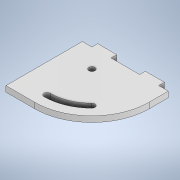
# Autodesk Inventor part: camMount
Saved by Autodesk Inventor 2020 (Build 240168000, 168)
## iProperties
Created: 2019-08-06
Part Number: camMount
Material: Generic
Document SubType Name: Modeling
Designer: n10208577
Density: 1 g/cm^3
Appearance: Default
Author: n10208577
Autodesk Inventor part; units mm, degrees
ref_plane "YZ Plane" through (0, 0, 0) normal (1, 0, 0) x (0, 1, 0)
ref_plane "XZ Plane" through (0, 0, 0) normal (0, 1, 0) x (-1, 0, 0)
ref_plane "XY Plane" through (0, 0, 0) normal (0, 0, 1) x (1, 0, 0)
sketch "Sketch1" plane through (0, 0, 0) normal (0, 1, 0) x (-1, 0, 0)
  arc A0 (9.7034, 16.3774) -> (9.7034, 19.5774) centre (9.7034, 17.9774) ccw
  circle A1 centre (9.7034, -5.5226) radius 1.6
  line L0 (9.7034, -15.5226) -> (-5.2966, -15.5226)
  line L1 (-15.2966, -15.5226) -> (-20.2966, -15.5226)
  line L2 (19.7034, -15.5226) -> (24.7034, -15.5226)
  line L3 (24.7034, -15.5226) -> (24.7034, 24.4774)
  line L4 (24.7034, 24.4774) -> (9.7034, 24.4774)
  arc A2 (-8.0449, 12.2258) -> (-5.7822, 9.963) centre (-6.9136, 11.0944) ccw
  arc A3 (9.7034, 16.3774) -> (-5.7822, 9.963) centre (9.7034, -5.5226) ccw
  arc A4 (9.7034, 19.5774) -> (-8.0449, 12.2258) centre (9.7034, -5.5226) ccw
  arc A5 (9.7034, 24.4774) -> (-20.2966, -5.5226) centre (9.7034, -5.5226) ccw
  line L5 (-20.2966, -15.5226) -> (-20.2966, -5.5226)
  line L6 (-15.2966, -15.5226) -> (-15.2966, -18.5226)
  line L7 (-15.2966, -18.5226) -> (-5.2966, -18.5226)
  line L8 (-5.2966, -18.5226) -> (-5.2966, -15.5226)
  line L9 (24.7034, -15.5226) -> (19.7034, -15.5226)
  line L10 (19.7034, -15.5226) -> (19.7034, -18.5226)
  line L11 (19.7034, -18.5226) -> (9.7034, -18.5226)
  line L12 (9.7034, -18.5226) -> (9.7034, -15.5226)
  point P0 (0, 0)
  constraints: 26 end point, 10 point on circle, 6 centre point
extrude "Extrusion1" add sketch "Sketch1" along normal blind 3
body "Solid1"
